2.5mm_top (Autodesk Fusion 360 design; units mm, degrees)
Autodesk Fusion 360 part; units mm, degrees
note: some values were not read from the file. Set by a fixed rule: which sketch regions a step uses.
sketch "Sketch1" plane through (0, 0, 0) normal (0, 1, 0) x (1, 0, 0)
  line L0 (0.0896, -1.2) -> (0.55, -1.2)
  line L1 (0.55, -1.2) -> (0.55, 0)
  line L2 (0.55, 0) -> (0, 0)
  line L3 (0, -0.845) -> (-0.25, -0.845)
  line L4 (-0.25, -0.845) -> (-0.25, -0.795)
  line L5 (-0.25, -0.795) -> (-0.75, -0.795)
  line L6 (-0.75, -0.795) -> (-0.75, -0.845)
  line L7 (-0.75, -0.845) -> (-2.6, -0.845)
  line L8 (-2.6, -0.845) -> (-2.9, -0.745)
  line L9 (-2.9, -0.745) -> (-2.9, -0.435)
  line L10 (-2.9, -0.435) -> (0, -0.435)
  line L11 (0, -0.435) -> (0, 0)
  line L12 (0, -0.845) -> (0.05, -0.845)
  line L13 (0.05, -0.845) -> (0.0125, -1.1112)
  line L14 (0.0896, -1.2) -> (0.0125, -1.1112)
  line L15 (0.0125, -1.1112) -> (0, -1.2) construction
  line L16 (0, -1.2) -> (0.0896, -1.2) construction
  point P0 (0, -1.2)
  point P1 (0, -1.2)
  dimension "d4" = 0.55
  dimension "d5" = 0.435
  dimension "d7" = 0.25
  dimension "d8" = 0.5
  dimension "d10" = 0.3
  dimension "d11" = 0.1
  dimension "d27" = 1.2
  dimension "d28" = 0.845
  dimension "d29" = 0.05
  dimension "d40" = 0.05
  dimension "d41" = 0.0896
  dimension "d42" = 0.0896
  dimension "d43" = 2.9
  constraint perpendicular L0 L1
  constraint coincident L2.end L11.end
  constraint perpendicular L3 L4
  constraint perpendicular L5 L6
  constraint perpendicular L6 L7
  constraint perpendicular L7 L9
  constraint perpendicular L6 L10
  constraint collinear L3 L7
  constraint coincident P0 L0
  constraint perpendicular L2 L11
  constraint perpendicular L11 L12
  constraint vertical L3.start P1
  constraint vertical L11
  constraint horizontal L3
  constraint coincident P0 L15.end
  constraint coincident P1 L13
  constraint vertical L10.end P1
  measures "d4" distance of P0 L0.end
  measures "d5" distance of L2.end L10
  measures "d7" distance of L3.start L3.end
  measures "d8" distance of L4.end L5.end
  measures "d10" horizontal distance of L7.end L8.end
  measures "d11" vertical distance of L7.end L8.end
  measures "d27" distance of L0 L2
  measures "d28" distance of L2.end L7
  measures "d29" distance of L5.end L6.end
  measures "d40" distance of L3.start L12.end
  measures "d41" distance of P1 L0.start
  measures "d42" distance of P1 L13.end
  measures "d43" distance of L9.end L10.end
revolve "Revolve1" add sketch "Sketch1" angle 360 about axis through (0.55, 0, 0) along (-1, 0, 0)
sketch "Sketch3" plane through (0.55, 0, 0) normal (1, 0, 0) x (0, 1, 0)
  circle A0 centre (0, 0) radius 1.2
  arc A1 (-0.7381, -0.9462) -> (-0.5709, -0.994) centre (-0.5946, -0.7606) ccw
  line L0 (-1.1216, 0.2358) -> (-1.0497, 0.0739)
  arc A2 (0.6387, -0.0616) -> (1.1792, 0.222) centre (0.9331, 0.0341) cw
  line L1 (-0.1223, 1.1393) -> (-0.2539, 1.0209)
  arc A3 (-1.0497, 0.0739) -> (-0.9743, -0.0197) centre (-0.8388, 0.1667) ccw
  arc A4 (0.0411, 1.199) -> (-0.1223, 1.1393) centre (0.0342, 0.9644) ccw
  arc A5 (1.1792, 0.222) -> (1.1533, 0.3311) centre (0.0001, -0.0004) ccw
  arc A6 (-0.4807, 0.4248) -> (-1.0847, 0.513) centre (-0.7752, 0.5204) cw
  line L2 (0.7767, 0.5881) -> (0.2557, 0.5882)
  line L3 (0.7687, -0.8504) -> (0.8056, -0.6773)
  arc A7 (-1.0847, 0.513) -> (-1.1278, 0.4095) centre (0, -0.0001) ccw
  arc A8 (-1.1278, 0.4095) -> (-1.1216, 0.2358) centre (-0.9069, 0.3304) ccw
  line L4 (-0.2824, -0.9328) -> (0.1391, -0.6266)
  arc A9 (0.8056, -0.6773) -> (0.7996, -0.5571) centre (0.5805, -0.6283) ccw
  arc A10 (-0.5526, -0.3261) -> (-0.8232, -0.8732) centre (-0.7346, -0.5766) cw
  arc A11 (0.6716, -0.9947) -> (0.7687, -0.8504) centre (0.5393, -0.8008) ccw
  arc A12 (0.8928, 0.5567) -> (0.7767, 0.5881) centre (0.7767, 0.3577) ccw
  arc A13 (0.5758, -1.053) -> (0.6716, -0.9947) centre (-0.0001, -0.0004) ccw
  arc A14 (-0.8232, -0.8732) -> (-0.7381, -0.9462) centre (-0.0001, -0.0002) ccw
  arc A15 (1.1533, 0.3311) -> (1.0461, 0.4681) centre (0.928, 0.2653) ccw
  arc A16 (0.2557, 0.5882) -> (0.1529, 1.1899) centre (0.2555, 0.8978) cw
  line L5 (0.7996, -0.5571) -> (0.6387, -0.0616)
  arc A17 (-0.2539, 1.0209) -> (-0.3197, 0.9202) centre (-0.1006, 0.849) ccw
  line L6 (-0.5709, -0.994) -> (-0.3948, -0.9757)
  line L7 (1.0461, 0.4681) -> (0.8928, 0.5567)
  line L8 (-0.9743, -0.0197) -> (-0.5526, -0.3261)
  arc A18 (0.1391, -0.6266) -> (0.5758, -1.053) centre (0.3211, -0.8771) cw
  line L9 (-0.3197, 0.9202) -> (-0.4807, 0.4248)
  arc A19 (-0.3948, -0.9757) -> (-0.2824, -0.9328) centre (-0.4178, -0.7464) ccw
  arc A20 (0.1529, 1.1899) -> (0.0411, 1.199) centre (0.0001, -0.0003) ccw
  circle A21 centre (0, 0) radius 1.1997
  constraint coincident A0.centre A21.centre
  constraint coincident A16.end A21
extrude "Extrude2" add sketch "Sketch3" along normal blind 1.05 contours A0 A1 L0 A2 L1 A3 A4 A5 A6 L2 L3 A7 A8 L4 A9 A10 A11 A12 A13 A14 A15 A16 L5 A17 L6 L7 L8 A18 L9 A19 A20 A21
move_body "Move1" bodies 1 to x (0, 0, 1) y (0, 1, 0) z (-1, 0, 0) at (0, 0, 0)
equation "d5 = ( 0.87 / 2 ) * 1 mm"
equation "d25 = 1.6 mm - 0.55 mm"
equation "d27 = ( 2.4 / 2 ) * 1 mm"
equation "d28 = ( var / 2 )"
equation "var = 1.690 mm"
equation "d42 = d41"
